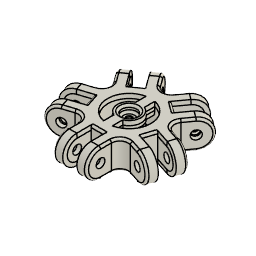
CenterRingV1_v14 (Autodesk Fusion 360 design; units mm, degrees)
Autodesk Fusion 360 part; units mm, degrees
sketch "Sketch1" plane through (0, 0, 0) normal (0, 0, 1) x (1, 0, 0)
  circle A0 centre (0, 0) radius 5.1
  circle A1 centre (0, 0) radius 7.5
  line L0 (0, 0) -> (0, -7.5) construction
  line L1 (0, -7.5) -> (1.6, -7.5) construction
  line L2 (0, -7.5) -> (-1.5, -7.5) construction
  line L3 (-1.5, -7.5) -> (-1.5, -7.3485)
  line L4 (1.6, -7.5) -> (1.6, -7.3273)
  line L5 (1.6, -7.5) -> (1.6, -14.25)
  line L6 (0, -7.5) -> (0, -9.25) construction
  line L7 (0, -9.25) -> (1.6, -9.25) construction
  line L8 (0, -9.25) -> (-1.5, -9.25) construction
  line L9 (0, -9.25) -> (0, -11.75) construction
  line L10 (1.6, -7.5) -> (-1.6, -7.5)
  line L11 (-1.6, -7.5) -> (-1.6, -14.25)
  line L12 (1.6, -14.25) -> (4, -14.25)
  line L13 (4, -14.25) -> (4, -6.3443)
  line L14 (-1.6, -14.25) -> (-4, -14.25)
  line L15 (-4, -14.25) -> (-4, -6.3443)
  dimension "d1" = 10.2
  dimension "d4" = 15
  dimension "d5" = 1.6
  dimension "d6" = 1.5
  dimension "d7" = 6.75
  dimension "d8" = 1.75
  dimension "d9" = 2.5
  dimension "d10" = 3.2
  dimension "d14" = 6.75
  constraint coincident A0.centre A1.centre
  constraint concentric A0 A1
  constraint coincident A1 L0.end
  constraint vertical L0
  constraint perpendicular L0 L1
  constraint perpendicular L0 L2
  constraint coincident A1 L3.end
  constraint perpendicular L2 L3
  constraint coincident A1 L4.end
  constraint perpendicular L1 L4
  constraint perpendicular L1 L5
  constraint coincident L5 L7.end
  constraint perpendicular L5 L7
  constraint perpendicular L7 L9
  constraint horizontal L10
  constraint vertical L11
  constraint perpendicular L5 L12
  constraint coincident A1 L13.end
  constraint perpendicular L12 L13
  constraint perpendicular L11 L14
  constraint coincident A1 L15.end
  constraint perpendicular L14 L15
  measures "d1" diameter of A0
  measures "d4" diameter of A1
  measures "d5" distance of L0.end L1.end
  measures "d6" distance of L0.end L2.end
  measures "d7" distance of L1.end L5.end
  measures "d8" distance of L0.end L6.end
  measures "d9" distance of L6.end L9.end
  measures "d10" distance of L1.end L10.end
  measures "d14" distance of L10.end L11.end
extrude "Extrude1" add sketch "Sketch1" along normal blind 6.75 makes body 1
sketch "Sketch2" plane through (-1.6, 0, 0) normal (1, 0, 0) x (0, 1, 0)
  line L0 (-14.25, 0) -> (-7.5, 0)
  line L1 (-7.5, 0) -> (-7.5, 6.75)
  line L2 (-7.5, 6.75) -> (-14.25, 6.75)
  line L3 (-14.25, 6.75) -> (-14.25, 0)
  line L4 (-14.25, 6.75) -> (-7.5, 6.75)
  line L5 (-7.5, 6.75) -> (-7.5, 0)
  line L6 (-7.5, 0) -> (-14.25, 0)
  line L7 (-14.25, 0) -> (-14.25, 6.75)
  line L8 (-14.25, 6.75) -> (-7.5, 0) construction
  circle A0 centre (-10.875, 3.375) radius 0.95
  circle A1 centre (-10.875, 3.375) radius 3.375
  dimension "d12" = 6.75
  dimension "d13" = 6.75
  dimension "d15" = 1.9
  constraint horizontal L4
  constraint vertical L5
  constraint horizontal L6
  constraint vertical L7
  constraint coincident L0.end L1.start
  constraint coincident L2.end L3.start
  constraint midpoint L8 A0.centre
  constraint concentric A0 A1
  constraint tangent L6 A1
  measures "d12" distance of L1.end L0.end
  measures "d13" distance of L2.end L1.end
  measures "d15" diameter of A0
extrude "Extrude2" cut sketch "Sketch2" along normal blind 14 and the other way blind 5 contours L0 L3 L6 L7 A1 | L2 L3 L4 L7 A1 | A0 bodies 1
chamfer "Chamfer3" distance 0.1 distance2 1 4 edges at (-4, -11.7607, 3.0315) (1.6, -11.7607, 3.0315) (-1.6, -11.7607, 3.7185) (4, -11.7607, 3.7185) measured on face at (-4, -7.5379, 3.375) measured on face at (1.6, -8.3083, 3.375) measured on face at (-1.6, -8.3083, 3.375) measured on face at (4, -7.5379, 3.375) tangent chain off on bodies 1
chamfer "Chamfer8" distance 0.1 distance2 1 3 edges at (-1.6, -9.1875, 6.75) (-1.6, -9.1875, 0) (-1.6, -14.25, 3.375) measured on face at (-3.2, -8.2398, 6.75) measured on face at (3.2, -8.2398, 0) measured on face at (-1.6, -8.275, 3.375) tangent chain off on bodies 1
chamfer "Chamfer9" distance 0.1 distance2 1 3 edges at (1.6, -9.1875, 6.75) (1.6, -14.25, 3.375) (1.6, -9.1875, 0) measured on face at (3.2, -8.2398, 6.75) measured on face at (1.6, -8.275, 3.375) measured on face at (1.6, -8.275, 3.375) tangent chain off on bodies 1
pattern_circular "C-Pattern1" count 5 over 360 about axis through (0, 0, 1.75) along (0, 0, 1) of bodies 1 makes body 2 at (6.8373, -5.6213, 0) makes body 3 at (7.459, 4.7656, 0) makes body 4 at (-2.2274, 8.5666, 0) makes body 5 at (-8.8356, 0.5289, 0)
combine "Combine1" operation add target body 5 tool bodies 2 1 4 3
fillet "Fillet1" radius 2 10 edges at (4, -6.3443, 3.375) (4.7977, -5.7647, 3.375) (6.9651, 2.7815, 3.375) (7.2698, 1.8437, 3.375) (-0.493, 7.4838, 3.375) (0.493, 7.4838, 3.375) (-6.9651, 2.7815, 3.375) (-7.2698, 1.8437, 3.375) (-4.7977, -5.7647, 3.375) (-4, -6.3443, 3.375) on bodies 5
sketch "Sketch3" plane through (0, 0, 6.75) normal (0, 0, 1) x (-1, 0, 0)
  circle A0 centre (0, 0) radius 5.1
  arc A1 (-8.0902, -4.33) -> (-9.0902, -1.2523) centre (-9.7082, -3.1544) ccw
  line L0 (-8.0902, -4.33) -> (-9.6282, -6.4469)
  line L1 (-9.6282, -6.4469) -> (-7.7675, -7.7988)
  line L2 (-5.7837, -5.0684) -> (-3.0331, -7.0669)
  line L3 (-5.0168, -9.7973) -> (-3.1561, -11.1492)
  line L4 (-3.1561, -11.1492) -> (-1.618, -9.0322)
  arc A2 (1.618, -9.0322) -> (-1.618, -9.0322) centre (0, -10.2078) ccw
  line L5 (1.618, -9.0322) -> (3.1561, -11.1492)
  line L6 (3.1561, -11.1492) -> (5.0168, -9.7973)
  line L7 (3.0331, -7.0669) -> (5.7837, -5.0684)
  line L8 (7.7675, -7.7988) -> (9.6282, -6.4469)
  line L9 (9.6282, -6.4469) -> (8.0902, -4.33)
  arc A3 (9.0902, -1.2523) -> (8.0902, -4.33) centre (9.7082, -3.1544) ccw
  line L10 (9.0902, -1.2523) -> (11.5788, -0.4437)
  line L11 (11.5788, -0.4437) -> (10.8681, 1.7438)
  line L12 (7.6583, 0.7008) -> (6.6076, 3.9344)
  line L13 (9.8174, 4.9774) -> (9.1067, 7.1648)
  line L14 (9.1067, 7.1648) -> (6.618, 6.3562)
  arc A4 (4, 8.2583) -> (6.618, 6.3562) centre (6, 8.2583) ccw
  line L15 (4, 8.2583) -> (4, 10.875)
  line L16 (4, 10.875) -> (1.7, 10.875)
  line L17 (1.7, 7.5) -> (-1.7, 7.5)
  line L18 (-1.7, 10.875) -> (-4, 10.875)
  line L19 (-4, 10.875) -> (-4, 8.2583)
  arc A5 (-6.618, 6.3562) -> (-4, 8.2583) centre (-6, 8.2583) ccw
  line L20 (-6.618, 6.3562) -> (-9.1067, 7.1648)
  line L21 (-9.1067, 7.1648) -> (-9.8174, 4.9774)
  line L22 (-6.6076, 3.9344) -> (-7.6583, 0.7008)
  line L23 (-10.8681, 1.7438) -> (-11.5788, -0.4437)
  line L24 (-11.5788, -0.4437) -> (-9.0902, -1.2523)
  circle A6 centre (0, 0) radius 15
  circle A7 centre (0, 0) radius 5
  line L25 (-7.7675, -7.7988) -> (-5.7837, -5.0684)
  line L26 (-3.0331, -7.0669) -> (-5.0168, -9.7973)
  line L27 (5.0168, -9.7973) -> (3.0331, -7.0669)
  line L28 (5.7837, -5.0684) -> (7.7675, -7.7988)
  line L29 (10.8681, 1.7438) -> (7.6583, 0.7008)
  line L30 (6.6076, 3.9344) -> (9.8174, 4.9774)
  line L31 (1.7, 10.875) -> (1.7, 7.5)
  line L32 (-1.7, 7.5) -> (-1.7, 10.875)
  line L33 (-9.8174, 4.9774) -> (-6.6076, 3.9344)
  line L34 (-7.6583, 0.7008) -> (-10.8681, 1.7438)
  dimension "d24" = 30
  dimension "d25" = 10
  constraint concentric A0 A6
  constraint concentric A6 A7
  measures "d24" diameter of A6
  measures "d25" diameter of A7
sketch "Sketch4" plane through (0, 0, 0) normal (0, 0, 1) x (-1, 0, 0)
  circle A0 centre (0, 0) radius 5.1
  arc A1 (-8.0902, -4.33) -> (-9.0902, -1.2523) centre (-9.7082, -3.1544) ccw
  line L0 (-8.0902, -4.33) -> (-9.6282, -6.4469)
  line L1 (-9.6282, -6.4469) -> (-7.7675, -7.7988)
  line L2 (-5.7837, -5.0684) -> (-3.0331, -7.0669)
  line L3 (-5.0168, -9.7973) -> (-3.1561, -11.1492)
  line L4 (-3.1561, -11.1492) -> (-1.618, -9.0322)
  arc A2 (1.618, -9.0322) -> (-1.618, -9.0322) centre (0, -10.2078) ccw
  line L5 (1.618, -9.0322) -> (3.1561, -11.1492)
  line L6 (3.1561, -11.1492) -> (5.0168, -9.7973)
  line L7 (3.0331, -7.0669) -> (5.7837, -5.0684)
  line L8 (7.7675, -7.7988) -> (9.6282, -6.4469)
  line L9 (9.6282, -6.4469) -> (8.0902, -4.33)
  arc A3 (9.0902, -1.2523) -> (8.0902, -4.33) centre (9.7082, -3.1544) ccw
  line L10 (9.0902, -1.2523) -> (11.5788, -0.4437)
  line L11 (11.5788, -0.4437) -> (10.8681, 1.7438)
  line L12 (7.6583, 0.7008) -> (6.6076, 3.9344)
  line L13 (9.8174, 4.9774) -> (9.1067, 7.1648)
  line L14 (9.1067, 7.1648) -> (6.618, 6.3562)
  arc A4 (4, 8.2583) -> (6.618, 6.3562) centre (6, 8.2583) ccw
  line L15 (4, 8.2583) -> (4, 10.875)
  line L16 (4, 10.875) -> (1.7, 10.875)
  line L17 (1.7, 7.5) -> (-1.7, 7.5)
  line L18 (-1.7, 10.875) -> (-4, 10.875)
  line L19 (-4, 10.875) -> (-4, 8.2583)
  arc A5 (-6.618, 6.3562) -> (-4, 8.2583) centre (-6, 8.2583) ccw
  line L20 (-6.618, 6.3562) -> (-9.1067, 7.1648)
  line L21 (-9.1067, 7.1648) -> (-9.8174, 4.9774)
  line L22 (-6.6076, 3.9344) -> (-7.6583, 0.7008)
  line L23 (-10.8681, 1.7438) -> (-11.5788, -0.4437)
  line L24 (-11.5788, -0.4437) -> (-9.0902, -1.2523)
  circle A6 centre (0, 0) radius 2.9
  line L25 (1.15, 5.2869) -> (-1.15, 5.2869)
  line L26 (-1.15, 5.2869) -> (-1.15, -5.2869)
  line L27 (-1.15, -5.2869) -> (1.15, -5.2869)
  line L28 (1.15, -5.2869) -> (1.15, 5.2869)
  line L29 (1.15, 5.2869) -> (-1.15, -5.2869) construction
  line L30 (-1.15, 5.2869) -> (1.15, -5.2869) construction
  line L31 (-7.7675, -7.7988) -> (-5.7837, -5.0684)
  line L32 (-3.0331, -7.0669) -> (-5.0168, -9.7973)
  line L33 (5.0168, -9.7973) -> (3.0331, -7.0669)
  line L34 (5.7837, -5.0684) -> (7.7675, -7.7988)
  line L35 (10.8681, 1.7438) -> (7.6583, 0.7008)
  line L36 (6.6076, 3.9344) -> (9.8174, 4.9774)
  line L37 (1.7, 10.875) -> (1.7, 7.5)
  line L38 (-1.7, 7.5) -> (-1.7, 10.875)
  line L39 (-9.8174, 4.9774) -> (-6.6076, 3.9344)
  line L40 (-7.6583, 0.7008) -> (-10.8681, 1.7438)
  circle A7 centre (0, 0) radius 5.1
  arc A8 (4, 8.2583) -> (6.618, 6.3562) centre (6, 8.2583) ccw
  line L41 (6.618, 6.3562) -> (9.1067, 7.1648)
  line L42 (9.1067, 7.1648) -> (9.8174, 4.9774)
  line L43 (9.8174, 4.9774) -> (6.6076, 3.9344)
  line L44 (6.6076, 3.9344) -> (7.6583, 0.7008)
  line L45 (7.6583, 0.7008) -> (10.8681, 1.7438)
  line L46 (10.8681, 1.7438) -> (11.5788, -0.4437)
  line L47 (11.5788, -0.4437) -> (9.0902, -1.2523)
  arc A9 (9.0902, -1.2523) -> (8.0902, -4.33) centre (9.7082, -3.1544) ccw
  line L48 (8.0902, -4.33) -> (9.6282, -6.4469)
  line L49 (9.6282, -6.4469) -> (7.7675, -7.7988)
  line L50 (7.7675, -7.7988) -> (5.7837, -5.0684)
  line L51 (5.7837, -5.0684) -> (3.0331, -7.0669)
  line L52 (3.0331, -7.0669) -> (5.0168, -9.7973)
  line L53 (5.0168, -9.7973) -> (3.1561, -11.1492)
  line L54 (3.1561, -11.1492) -> (1.618, -9.0322)
  arc A10 (1.618, -9.0322) -> (-1.618, -9.0322) centre (0, -10.2078) ccw
  line L55 (-1.618, -9.0322) -> (-3.1561, -11.1492)
  line L56 (-3.1561, -11.1492) -> (-5.0168, -9.7973)
  line L57 (-5.0168, -9.7973) -> (-3.0331, -7.0669)
  line L58 (-3.0331, -7.0669) -> (-5.7837, -5.0684)
  line L59 (-5.7837, -5.0684) -> (-7.7675, -7.7988)
  line L60 (-7.7675, -7.7988) -> (-9.6282, -6.4469)
  line L61 (-9.6282, -6.4469) -> (-8.0902, -4.33)
  arc A11 (-8.0902, -4.33) -> (-9.0902, -1.2523) centre (-9.7082, -3.1544) ccw
  line L62 (-9.0902, -1.2523) -> (-11.5788, -0.4437)
  line L63 (-11.5788, -0.4437) -> (-10.8681, 1.7438)
  line L64 (-10.8681, 1.7438) -> (-7.6583, 0.7008)
  line L65 (-7.6583, 0.7008) -> (-6.6076, 3.9344)
  line L66 (-6.6076, 3.9344) -> (-9.8174, 4.9774)
  line L67 (-9.8174, 4.9774) -> (-9.1067, 7.1648)
  line L68 (-9.1067, 7.1648) -> (-6.618, 6.3562)
  arc A12 (-6.618, 6.3562) -> (-4, 8.2583) centre (-6, 8.2583) ccw
  line L69 (-4, 8.2583) -> (-4, 10.875)
  line L70 (-4, 10.875) -> (-1.7, 10.875)
  line L71 (-1.7, 10.875) -> (-1.7, 7.5)
  line L72 (-1.7, 7.5) -> (1.7, 7.5)
  line L73 (1.7, 7.5) -> (1.7, 10.875)
  line L74 (1.7, 10.875) -> (4, 10.875)
  line L75 (4, 10.875) -> (4, 8.2583)
  dimension "d31" = 5.8
  dimension "d32" = 2.3
  constraint coincident A0.centre A6.centre
  constraint horizontal L25
  constraint perpendicular L25 L26
  constraint parallel L25 L27
  constraint parallel L26 L28
  constraint coincident L29 A0.centre
  constraint coincident L30 A0.centre
  measures "d31" diameter of A6
  measures "d32" distance of L26.end L27.end
extrude "Extrude3" add sketch "Sketch4" along normal blind 6.75 contours A0 A6 L26 L28 A7 | A0 A6 L26 L28 A7 | A6 L26 L28 | A6 L28 | A6 L26 bodies 5
extrude "Extrude6" cut sketch "Sketch4" along normal blind 4 contours A0 A6 L26 L28 A7 | A0 A6 L26 L28 A7 | A6 L26 L28 | A6 L28 | A6 L26 bodies 5
hole "Hole1" at (0, 0, 6.75) direction (0, 0, -1) diameter 1.5 depth 4.5 tip angle 118 counterbore diameter 3.6 counterbore depth 1.5 bodies 5
chamfer "Chamfer2" distance 0.1 distance2 1 1 edges at (-0.6992, -0.2712, 4) measured on face at (0, 3.4748, 4) tangent chain off on bodies 5
chamfer "Chamfer4" distance 0.1 distance2 1 2 edges at (5.1, 0, 6.75) (-5.1, 0, 6.75) measured on face at (6.3801, -2.0451, 6.75) measured on face at (6.3801, -2.0451, 6.75) tangent chain off on bodies 5
chamfer "Chamfer5" distance 1 distance2 0.1 1 edges at (0.2846, 5.0921, 0) measured on face at (-1.6385, -4.8296, 3.25) tangent chain off on bodies 5
chamfer "Chamfer6" distance 0.1 distance2 1 6 edges at (-1.15, 3.8667, 6.75) (-2.9, 0, 6.75) (-1.15, -3.8667, 6.75) (1.15, -3.8667, 6.75) (2.9, 0, 6.75) (1.15, 3.8667, 6.75) measured on face at (4.0184, 5.4013, 6.75) measured on face at (4.0184, 5.4013, 6.75) measured on face at (4.0184, 5.4013, 6.75) measured on face at (4.0184, 5.4013, 6.75) measured on face at (4.0184, 5.4013, 6.75) measured on face at (4.0184, 5.4013, 6.75) tangent chain off on bodies 5
chamfer "Chamfer7" distance 1 distance2 0.1 7 edges at (-1.15, 3.8154, 4) (-1.15, -3.8154, 4) (-2.9, 0, 4) (-1.15, 3.8154, 4) (1.15, 3.8154, 4) (2.9, 0, 4) (1.15, -3.8154, 4) measured on face at (-1.15, 4.1998, 4.5833) measured on face at (-1.15, -3.431, 4.5833) measured on face at (-1.4022, 2.5385, 5.1667) measured on face at (-1.15, 4.1998, 4.5833) measured on face at (1.15, 3.431, 5.1667) measured on face at (1.4022, 2.5385, 4.5833) measured on face at (1.15, -3.431, 5.1667) tangent chain off on bodies 5
fillet "Fillet2" radius 0.5 1 edges at (-1.6782, 0.6509, 6.75) on bodies 5
fillet "Fillet3" radius 0.5 1 edges at (-1.6782, 0.6509, 5.25) on bodies 5
fillet "Fillet4" radius 0.5 40 edges at (4.8244, -6.6403, 6.75) (7.8624, -6.7605, 6.75) (12.3165, -8.2077, 3.375) (7.8624, -6.7605, 0) (4.8244, -6.6403, 0) (4, -9.5666, 0) (4, -14.25, 3.375) (4, -9.5666, 6.75) (11.612, 9.1774, 3.375) (8.8592, 5.3884, 0) (7.8061, 2.5364, 0) (10.3345, 0.848, 0) (14.7886, -0.5993, 3.375) (10.3345, 0.848, 6.75) (7.8061, 2.5364, 6.75) (8.8592, 5.3884, 6.75) (-5.1399, 13.8796, 3.375) (-2.3871, 10.0907, 0) (0, 8.2078, 0) (2.3871, 10.0907, 0) (5.1399, 13.8796, 3.375) (2.3871, 10.0907, 6.75) (0, 8.2078, 6.75) (-2.3871, 10.0907, 6.75) (-8.8592, 5.3884, 6.75) (-11.612, 9.1774, 3.375) (-8.8592, 5.3884, 0) (-7.8061, 2.5364, 0) (-10.3345, 0.848, 0) (-14.7886, -0.5993, 3.375) (-10.3345, 0.848, 6.75) (-7.8061, 2.5364, 6.75) (-7.8624, -6.7605, 6.75) (-12.3165, -8.2077, 3.375) (-7.8624, -6.7605, 0) (-4.8244, -6.6403, 0) (-4, -9.5666, 0) (-4, -14.25, 3.375) (-4, -9.5666, 6.75) (-4.8244, -6.6403, 6.75) on bodies 5
fillet "Fillet5" radius 0.5 10 edges at (-4.4084, 6.0676, 6.75) (-7.1329, -2.3176, 6.75) (4.4084, 6.0676, 6.75) (7.1329, -2.3176, 6.75) (0, -7.5, 6.75) (0, -7.5, 0) (7.1329, -2.3176, 0) (4.4084, 6.0676, 0) (-4.4084, 6.0676, 0) (-7.1329, -2.3176, 0) on bodies 5
